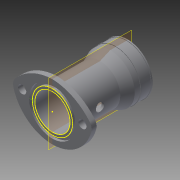
# Autodesk Inventor part: throttle_ETC
Saved by Autodesk Inventor 2015 (Build 190159000, 159)
## iProperties
Created: 2015-04-14
Part Number: throttle_ETC
Material: Generic
Description: insert part description/title
Document SubType Name: Modeling
Designer: frank
Density: 1 g/cm^3
Appearance: Default
Part Category: insert part category here and press enter to fill value
Author: frank
Autodesk Inventor part; units mm, degrees
ref_plane "XZ Plane" through (0, 0, 0) normal (0, 1, 0) x (-1, 0, 0)
ref_plane "XY Plane" through (0, 0, 0) normal (0, 0, 1) x (1, 0, 0)
sketch "Sketch1" plane through (0, 0, 0) normal (0, 0, 1) x (1, 0, 0)
  line L0 (14, -60) -> (14, -21.5)
  line L1 (14, -21.5) -> (17.5, -13.5)
  line L2 (17.5, -13.5) -> (17.5, 0)
  line L3 (19.5, -13.9184) -> (16, -21.9184)
  line L4 (16, -21.9184) -> (16, -60)
  line L5 (19.5, 0) -> (17.5, 0)
  line L6 (16, -60) -> (14, -60)
  line L7 (19.5, -1) -> (19.9, -1)
  line L8 (19.9, -1) -> (19.9, 0)
  line L9 (19.9, 0) -> (19.5, 0)
  line L10 (19.5, -8.5) -> (19.9, -8.5)
  line L11 (19.9, -8.5) -> (19.9, -9.5)
  line L12 (19.9, -9.5) -> (19.5, -9.5)
  line L13 (19.5, -9.5) -> (19.5, -13.9184)
  line L14 (19.5, -1) -> (19.5, -8.5)
  line L15 (0, 0) -> (0, -57.1164)
  point P0 (16, -38.699)
  dimension "d0" = 17.5
  dimension "d1" = 13.5
  dimension "d2" = 21.5
  dimension "d3" = 14
  dimension "d4" = 60
  dimension "d5" = 2
  dimension "d6" = 0.4
  dimension "d7" = 1
  dimension "d8" = 0.4
  dimension "d9" = 1
  dimension "d10" = 8.5
  constraints: 32 end point, 3 parallel, 2 coincident, 2 horizontal, 2 perpendicular, 2 point on line, 1 collinear, 1 vertical, 1 other
  measures "d0" distance of L15.start L2.end
  measures "d1" distance of L1.end L2.end
  measures "d2" vertical distance of L0.end L2.end
  measures "d3" distance from line of L15.start L0
  measures "d4" vertical distance of L2.end L0.start
  measures "d5" distance between parallel lines of L1 L3
  measures "d6" distance of L7.start L7.end
  measures "d7" distance of L7.end L8.end
  measures "d8" distance of L11.end L12.end
  measures "d9" distance of L10.end L11.end
  measures "d10" distance between parallel lines of L9 L10
revolve "Revolution1" add sketch "Sketch1" angle 360 about axis through (0, 0, 0) along (0, -1, 0)
sketch "Sketch5" plane through (0, -60, 0) normal (0, -1, 0) x (1, 0, 0)
  circle A0 centre (0, 0) radius 14 projected
  circle A1 centre (0, 0) radius 16 projected
  point P0 (-16, 0)
  constraints: 1 horizontal alignment, 1 other
sketch "Sketch6" plane through (0, 0, 0) normal (1, 0, 0) x (0, 1, 0)
  line L0 (0, 0) -> (-76, 0)
  line L1 (-21.9184, 16) -> (-60, 16) projected
  line L2 (0, 19.9) -> (0, -19.9) projected
  line L3 (-21.9184, -16) -> (-60, -16) projected
  line L4 (-1, -19.5) -> (-8.5, -19.5) projected
  line L5 (-40.9592, 16) -> (-40.9592, -16) construction
  circle A0 centre (-38, 0) radius 3.25
  line L6 (-60, 16) -> (-60, -16) projected
  dimension "d21" = 6.5
  dimension "d40" = 22
  constraints: 4 end point, 4 midpoint, 3 coincident, 1 centre point, 1 horizontal
  measures "d21" diameter of A0
  measures "d40" distance from line of L6 point (-38, 0)
extrude "Extrusion1" cut sketch "Sketch6" along normal through all both and the other way through all
sketch "Sketch7" plane through (0, -60, 0) normal (0, -1, 0) x (1, 0, 0)
  circle A0 centre (0, 0) radius 14 projected
  circle A1 centre (-24, 3.4731) radius 3.25
  circle A2 centre (24, 3.4731) radius 3.25
  circle A3 centre (0, 0) radius 18.5
  arc A4 (-29.548, 8.1402) -> (-31.0133, 1.6358) centre (-24, 3.4731) ccw
  arc A5 (-31.0133, 1.6358) -> (0, -22.5) centre (0.2614, 9.8292) ccw
  arc A6 (0, 22.5) -> (-29.548, 8.1402) centre (1.3447, -17.8473) ccw
  line L0 (-34.5214, 0) -> (40.2242, 0) construction
  circle A7 centre (0, 0) radius 14 construction
  line L1 (0, -32.9352) -> (0, 39.8381)
  arc A8 (31.0133, 1.6358) -> (29.548, 8.1402) centre (24, 3.4731) ccw
  arc A9 (0, -22.5) -> (31.0133, 1.6358) centre (-0.2614, 9.8292) ccw
  arc A10 (29.548, 8.1402) -> (0, 22.5) centre (-1.3447, -17.8473) ccw
  point P0 (0, -18.5)
  dimension "d28" = 37
  dimension "d24" = 6.5
  dimension "d25" = 48
  dimension "d26" = 7
  dimension "d27" = 6.5
  dimension "d29" = 0
  dimension "d30" = 0
  dimension "d31" = 4
  dimension "d33" = 22.5
  dimension "d34" = 4
  constraints: 12 point on circle, 8 centre point, 5 symmetric about line, 4 end point, 2 tangent, 1 horizontal, 1 vertical, 1 vertical alignment, 6 other
  measures "d24" diameter of A2
  measures "d25" distance of A2.centre A1.centre
  measures "d27" diameter of A1
  measures "d29" distance of A1.centre A4.centre
  measures "d30" distance of A1.centre A4.centre
  measures "d31" radial gap between concentric circles of A1 A4
  measures "d33" distance of A6.start point (0, 0)
  measures "d34" distance of point (0, -18.5) A5.end
extrude "Extrusion2" add sketch "Sketch7" against normal blind 4 contours A0 L1 A3 | A0 L1 A3 | L1 A10 A8 A9 A3 | A3 L1 A5 A4 A6
sketch "Sketch8" plane through (0.2614, -60, 9.8292) normal (0, -1, 0) x (0.789176, 0, -0.6141671)
  circle A0 centre (5.8304, -7.9175) radius 16
  circle A1 centre (5.8304, -7.9175) radius 18.5 projected
  circle A2 centre (5.8304, -7.9175) radius 18.5
  constraints: 2 centre point, 2 coincident, 1 concentric
extrude "Extrusion3" cut sketch "Sketch8" against normal blind 2
fillet "Fillet1" radius 2 1 edges at (-16, -56, 0)
body "Solid1"
